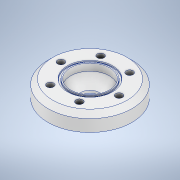
# Autodesk Inventor part: ODSY-0003-202
Saved by Autodesk Inventor 2021 (Build 250183000, 183)
## iProperties
Company: ERPL
Created: 2021-10-02
Part Number: ODSY-0003-202
Material: Aluminum 6061
Document SubType Name: Modeling
Designer: WYATT ROBINSON
Density: 2.7 g/cm^3
Appearance: Aluminum - Flat
Mass: 187.01 g
Surface Area: 174.96 cm^2
Volume: 69.263 cm^3
Project: ODYSSEY
Description: INJECTOR SPACER
Author: WYATT ROBINSON
Revision Number: 00
Autodesk Inventor part; units mm, degrees
ref_plane "YZ Plane" through (0, 0, 0) normal (1, 0, 0) x (0, 1, 0)
ref_plane "XZ Plane" through (0, 0, 0) normal (0, 1, 0) x (-1, 0, 0)
ref_plane "XY Plane" through (0, 0, 0) normal (0, 0, 1) x (1, 0, 0)
sketch "Sketch1" plane through (0, 0, 0) normal (0, 0, 1) x (1, 0, 0)
  line L0 (9.525, 0) -> (19.05, 0)
  line L1 (41.275, 19.05) -> (19.05, 19.05)
  line L2 (19.05, 19.05) -> (19.05, 12.065)
  line L3 (19.05, 12.065) -> (9.525, 2.54)
  line L4 (9.525, 2.54) -> (9.525, 0)
  line L5 (0, -3.81) -> (0, 22.86) projected
  line L6 (19.05, 0) -> (19.05, 2.54)
  line L7 (19.05, 2.54) -> (41.275, 2.54)
  line L8 (41.275, 2.54) -> (41.275, 19.05)
  point P0 (0, 0)
  dimension "d37" = 45
  dimension "d40" = 2.54
  dimension "d57" = 19.05
  dimension "d58" = 9.525
  dimension "d59" = 19.05
  dimension "d60" = 41.275
  dimension "d61" = 2.54
  dimension "d62" = 19.05
  constraints: 16 end point, 3 perpendicular, 2 vertical, 1 horizontal, 1 point on line
  measures "d37" angle of L2 L3
  measures "d40" distance of L3.end L0.start
  measures "d57" distance between parallel lines of L5 L2
  measures "d58" distance from line of point (0, 0) L4
  measures "d59" distance between parallel lines of L5 L6
  measures "d60" distance between parallel lines of L5 L8
  measures "d61" distance of L0.end L6.end
  measures "d62" distance between parallel lines of L0 L1
revolve "Revolution1" add sketch "Sketch1" angle 360 about axis through (0, -10, 0) along (0, 1, 0)
sketch "Sketch4" plane through (0, 0, 0) normal (0, -1, 0) x (1, 0, 0)
  point P0 (0, 0)
  point P1 (-28.575, 0)
  dimension "d50" = 28.575
  constraints: 1 horizontal alignment
  measures "d50" distance of point (0, 0) point (-28.575, 0)
hole "Hole2" at (-28.575, 0, 0) direction (0, 1, 0) diameter 6.7564 end through all clearance for "Socket Head Cap Screw" size "1/4" standard "Ansi Unified Screw Threads"
pattern_circular "Circular Pattern3" count 6 over 360 about axis through (0, 1.27, 0) along (0, -1, 0) of "Hole2"
chamfer "Chamfer3" distance 4.7625 angle 45 1 edges at (-41.275, 19.05, 0)
sketch "Sketch8" plane through (0, 0, 0) normal (0, 0, 1) x (1, 0, 0)
  line L0 (-22.2758, 19.05) -> (-20.1422, 19.05)
  line L1 (-20.1422, 19.05) -> (-20.1422, 18.034)
  line L2 (-20.3962, 17.78) -> (-22.0218, 17.78)
  line L3 (-22.2758, 18.034) -> (-22.2758, 19.05)
  line L4 (0, -5.1288) -> (0, 30.7731) projected
  arc A0 (-22.2758, 18.034) -> (-22.0218, 17.78) centre (-22.0218, 18.034) ccw
  arc A1 (-20.3962, 17.78) -> (-20.1422, 18.034) centre (-20.3962, 18.034) ccw
  line L5 (-19.05, 19.05) -> (19.05, 19.05) projected
  point P0 (0, 0)
  point P1 (-22.2758, 17.78)
  dimension "d88" = 1.27
  dimension "d90" = 22.2758
  dimension "d91" = 2.1336
  dimension "d92" = 0.254
  dimension "d93" = 0.254
  dimension "d94" = 0
  constraints: 8 end point, 4 point on circle, 4 tangent, 2 centre point, 2 parallel, 2 point on line, 1 horizontal, 1 perpendicular
  measures "d88" distance of point (-22.276, 17.78) L0.start
  measures "d90" distance between parallel lines of L4 L3
  measures "d91" distance of L0.start L0.end
  measures "d92" radius of A0
  measures "d93" radius of A1
  measures "d94" distance between parallel lines of L5 L0
revolve "Revolution5" cut sketch "Sketch8" angle 360 about axis through (0, -10, 0) along (0, 1, 0)
sketch "Sketch9" plane through (0, 0, 0) normal (0, 0, 1) x (1, 0, 0)
  line L0 (-14.8717, 1.27) -> (-13.2461, 1.27)
  line L1 (-12.9921, 1.016) -> (-12.9921, 0)
  line L2 (-12.9921, 0) -> (-15.1257, 0)
  line L3 (-15.1257, 0) -> (-15.1257, 1.016)
  arc A0 (-14.8717, 1.27) -> (-15.1257, 1.016) centre (-14.8717, 1.016) ccw
  arc A1 (-12.9921, 1.016) -> (-13.2461, 1.27) centre (-13.2461, 1.016) ccw
  line L4 (0, -3.81) -> (0, 22.86) projected
  line L5 (0, -15.7794) -> (0, 28.2703) construction
  point P0 (0, 0)
  dimension "d96" = 15.1257
  dimension "d97" = 0.254
  dimension "d98" = 1.27
  dimension "d99" = 2.1336
  constraints: 10 end point, 4 point on circle, 4 tangent, 2 centre point, 2 parallel, 2 point on line, 1 equal radius, 1 horizontal, 1 perpendicular, 1 vertical
  measures "d96" distance from line of point (0, 0) L3
  measures "d97" radius of A0
  measures "d98" distance between parallel lines of L2 L0
  measures "d99" distance of L1.end L2.end
revolve "Revolution6" cut sketch "Sketch9" angle 360 about axis through (0, -10, 0) along (0, 1, 0)
body "Solid1"
